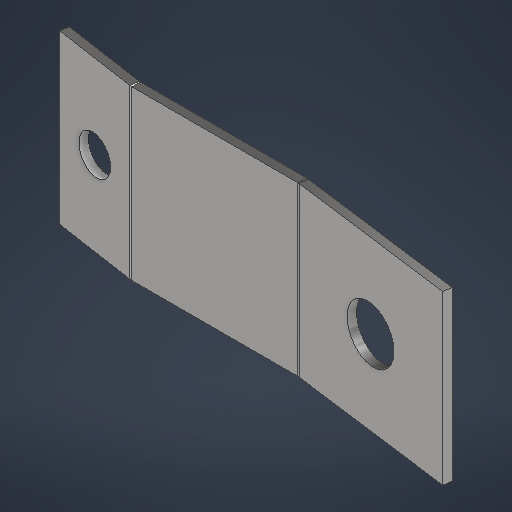
# Autodesk Inventor part: Pressure platform
Saved by Autodesk Inventor 2026.3 (Build 303398000, 398)
## iProperties
Created: 2026-08-04
Part Number: Pressure platform
Material: Generic
Document SubType Name: Sheet Metal
Designer: matot
Density: 1 g/cm^3
Sheet Metal Rule: Default_mm
Appearance: Default
Author: matot
Autodesk Inventor part; units mm, degrees
ref_plane "YZ Plane" through (0, 0, 0) normal (1, 0, 0) x (0, 1, 0)
ref_plane "XZ Plane" through (0, 0, 0) normal (0, 1, 0) x (-1, 0, 0)
ref_plane "XY Plane" through (0, 0, 0) normal (0, 0, 1) x (1, 0, 0)
sketch "Sketch1" plane through (0, 0, 0) normal (0, 0, 1) x (1, 0, 0)
  line L0 (-18, 8) -> (32, 8)
  line L1 (32, 8) -> (32, -12)
  line L2 (32, -12) -> (-18, -12)
  line L3 (-18, -12) -> (-18, 8)
  point P0 (0, 0)
  dimension "d0" = 50
  dimension "d1" = 20
  measures "d0" distance of L0.start L0.end
  measures "d1" distance of L2.end L0.start
extrude "Plate1" add sketch "Sketch1" along normal blind 1
sketch "Sketch2" plane through (0, 0, 1) normal (0, 0, 1) x (1, 0, 0)
  line L0 (32, 8) -> (-18, 8) projected
  line L1 (12, 8) -> (12, -12)
  line L2 (-18, -12) -> (32, -12) projected
  line L3 (32, -12) -> (-18, -12) projected
  line L4 (32, 8) -> (32, -12) projected
  point P0 (0, 0)
  dimension "d3" = 20
  constraints: 2 end point, 2 point on line, 1 perpendicular, 1 vertical
  measures "d3" distance between parallel lines of L4 L1
fold "Fold1" angle 7.5 bend radius 1 thickness 1 k factor 0.44 line from (12, 8, 1) to (12, -12, 1) line at bend centre moving side (1, 0, 0) folds toward (0, 0, 1)
sketch "Sketch4" plane through (31.7717, -12, 3.6068) normal (-0.1305262, 0, 0.9914449) x (0.9914449, 0, 0.1305262)
  line L0 (0, 20) -> (0, 0) projected
  line L1 (0, 0) -> (-19.9058, 0) projected
  point P0 (-31.9707, 12)
  point P1 (-10, 10)
  point P2 (0, 10)
  dimension "d10" = 10
  dimension "d11" = 10
  constraints: 1 midpoint
  measures "d10" distance of point (0, 10) point (-10, 10)
  measures "d11" distance from line of L1 point (-10, 10)
hole "Hole1" at (21.8573, -2, 2.3015) direction (0.1305262, 0, -0.9914449) diameter 6.5 end through all
sketch "Sketch5" plane through (0, 0, 0) normal (0, 0, -1) x (-1, 0, 0)
  line L0 (18, 8) -> (-11.9058, 8) projected
  line L1 (8, 8) -> (8, -12)
  line L2 (18, 8) -> (18, -12) projected
  line L3 (18, -12) -> (-11.9058, -12) projected
  point P0 (0, 0)
  dimension "d19" = 20
  dimension "d20" = 10
  constraints: 2 end point, 1 perpendicular, 1 point on line, 1 vertical
  measures "d19" distance of L1.start L1.end
  measures "d20" distance between parallel lines of L2 L1
fold "Fold2" angle 8.5 bend radius 1 thickness 1 k factor 0.44 line from (-8, 8, 0) to (-8, -12, 0) line at bend centre moving side (-1, 0, 0) folds toward (0, 0, -1)
sketch "Sketch6" plane through (-17.9733, -12, -0.4843) normal (-0.1478094, 0, 0.9890159) x (0.9890159, 0, 0.1478094)
  line L0 (9.8932, 0) -> (0, 0) projected
  line L1 (9.8932, 0) -> (9.8932, 20) projected
  line L2 (0, 0) -> (0, 20) projected
  point P0 (17.8475, 12)
  point P1 (4.9467, 10)
  point P2 (0, 10)
  dimension "d27" = 10
  dimension "d28" = 4.9465
  dimension "d29" = 9.8932
  constraints: 1 midpoint
  measures "d27" distance from line of L0 point (4.947, 10)
  measures "d28" distance from line of point (4.947, 10) L1
  measures "d29" distance from line of point (0, 10) L1
hole "Hole2" at (-13.081, -2, 0.2469) direction (0.1478094, 0, -0.9890159) diameter 4.5 end through all
equation "\"d2\" = Thickness"
equation "\"d4\" = BendReliefWidth"
equation "\"d5\" = BendReliefDepth"
equation "\"d6\" = MinimumRemnant"
equation "\"d7\" = TransitionRadius"
equation "\"d9\" = BendRadius"
equation "\"d17\" = Thickness"
equation "\"d21\" = BendReliefWidth"
equation "\"d22\" = BendReliefDepth"
equation "\"d23\" = MinimumRemnant"
equation "\"d24\" = TransitionRadius"
equation "\"d26\" = BendRadius"
equation "\"BendRadius\" = Thickness"
equation "\"BendReliefWidth\" = Thickness"
equation "\"BendReliefDepth\" = 0.5 * Thickness"
equation "\"CornerReliefSize\" = 4 * Thickness"
equation "\"MinimumRemnant\" = 2 * Thickness"
equation "\"TransitionRadius\" = BendRadius"
equation "\"JacobiRadiusSize\" = BendRadius"
equation "\"GapSize\" = Thickness"
equation "\"Thickness\" = 1"
body "Solid1"
